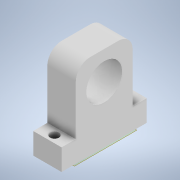
# Autodesk Inventor part: motor_mount_wrist
Saved by Autodesk Inventor 2022 (Build 260153000, 153)
## iProperties
Created: 2022-01-26
Part Number: motor_mount_wrist
Material: Generic
Document SubType Name: Modeling
Designer: pauly
Density: 1 g/cm^3
Appearance: Default
Author: pauly
Autodesk Inventor part; units mm, degrees
ref_plane "YZ Plane" through (0, 0, 0) normal (1, 0, 0) x (0, 1, 0)
ref_plane "XZ Plane" through (0, 0, 0) normal (0, 1, 0) x (-1, 0, 0)
ref_plane "XY Plane" through (0, 0, 0) normal (0, 0, 1) x (1, 0, 0)
sketch "Sketch1" plane through (0, 0, 0) normal (1, 0, 0) x (0, 1, 0)
  line L0 (0, 0) -> (63.5, 0)
  line L1 (76.2, -12.7) -> (76.2, -38.1)
  line L2 (63.5, -50.8) -> (0, -50.8)
  line L3 (0, -50.8) -> (0, 0)
  circle A0 centre (50.8, -25.4) radius 16.002
  arc A1 (76.2, -12.7) -> (63.5, 0) centre (63.5, -12.7) ccw
  arc A2 (63.5, -50.8) -> (76.2, -38.1) centre (63.5, -38.1) ccw
  point P0 (76.2, -50.8)
  point P1 (76.2, 0)
  dimension "d1" = 76.2
  dimension "d2" = 50.8
  dimension "d6" = 32.004
  dimension "d7" = 12.7
  constraints: 8 end point, 4 point on circle, 4 point on line, 4 tangent, 3 centre point, 2 parallel, 1 equal radius, 1 horizontal, 1 perpendicular
  measures "d1" distance of point (76.2, -50.8) L2.end
  measures "d2" distance of point (76.2, 0) point (76.2, -50.8)
  measures "d6" diameter of A0
  measures "d7" radius of A1
extrude "Extrusion1" add sketch "Sketch1" along normal blind 25.4
ref_plane "Work Plane1" through (0, 0, -50.8) normal (0, -1, 0) x (1, 0, 0)
sketch "Sketch2" plane through (0, 0, -50.8) normal (0, -1, 0) x (1, 0, 0)
  line L0 (0, 50.8) -> (25.4, 50.8)
  line L1 (25.4, 50.8) -> (25.4, 63.5)
  line L2 (25.4, 63.5) -> (0, 63.5)
  line L3 (0, 63.5) -> (0, 50.8)
  line L4 (0, 50.8) -> (0, 0) projected
  line L5 (0, 0) -> (25.4, 0)
  line L6 (25.4, 0) -> (25.4, -12.7)
  line L7 (25.4, -12.7) -> (0, -12.7)
  line L8 (0, -12.7) -> (0, 0)
  circle A0 centre (12.7, 57.15) radius 3.9687
  circle A1 centre (12.7, -6.35) radius 3.9688
  dimension "d11" = 25.4
  dimension "d12" = 25.4
  dimension "d13" = 12.7
  dimension "d14" = 12.7
  dimension "d15" = 7.9375
  dimension "d16" = 7.9375
  constraints: 16 end point, 4 parallel, 2 centre point, 2 horizontal, 2 perpendicular
  measures "d11" distance of L2.end L1.end
  measures "d12" distance of L6.end L7.end
  measures "d13" distance of L0.end L1.end
  measures "d14" distance of L7.end L4.end
  measures "d15" diameter of A0
  measures "d16" diameter of A1
extrude "Extrusion2" add sketch "Sketch2" against normal blind 19.05 contours L3 L2 L1 L0 | L5 L6 L7 L8 | A0 | A1
sketch "Sketch3" plane through (0, 19.05, -50.8) normal (0, 1, 0) x (1, 0, 0)
  line L0 (0, -63.5) -> (25.4, -63.5) projected
  circle A0 centre (12.7, -57.15) radius 3.9688
  line L1 (25.4, 12.7) -> (0, 12.7) projected
  circle A1 centre (12.7, 6.35) radius 3.9688
  point P0 (0, -50.8)
  dimension "d20" = 7.9375
  constraints: 2 centre point
  measures "d20" diameter of A0
hole "Hole1" at (12.7, 19.05, -57.15) direction (0, -1, 0) diameter 6.4008 end through all counterbore diameter 7.9375 counterbore depth 6.35 thread size "5/16-18 UNC" class "2B" standard "ANSI Unified Screw Threads"
hole "Hole2" at (12.7, 19.05, 6.35) direction (0, -1, 0) diameter 6.4008 end through all counterbore diameter 7.9375 counterbore depth 6.35 thread size "5/16-18 UNC" class "2B" standard "ANSI Unified Screw Threads"
equation "\"d23\" = d12"
equation "\"d30\" = d12"
body "Solid1"
